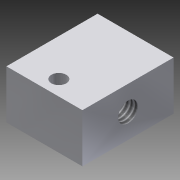
# Autodesk Inventor part: T2.5 belt holder
Saved by Autodesk Inventor 2015 SP1 (Build 190203100, 203)
## iProperties
Created: 2015-04-24
Part Number: T2.5 belt holder
Material: Aluminum 6061
Document SubType Name: Modeling
Designer: ubik
Density: 2.7 g/cm^3
Appearance: Aluminum - Flat
Author: ubik
Autodesk Inventor part; units mm, degrees
ref_plane "YZ Plane" through (0, 0, 0) normal (1, 0, 0) x (0, 1, 0)
ref_plane "XZ Plane" through (0, 0, 0) normal (0, 1, 0) x (-1, 0, 0)
ref_plane "XY Plane" through (0, 0, 0) normal (0, 0, 1) x (1, 0, 0)
sketch "Sketch1" plane through (0, 0, 0) normal (0, 0, 1) x (1, 0, 0)
  line L0 (3.9408, -0.7944) -> (3.5592, -0.7944)
  line L1 (1.4408, -0.7944) -> (1.0592, -0.7944)
  line L2 (-1.0592, -0.7944) -> (-1.4408, -0.7944)
  line L3 (-3.5592, -0.7944) -> (-3.9408, -0.7944)
  line L4 (-6.0592, -0.7944) -> (-6.25, -0.7944)
  line L5 (6.25, -0.7944) -> (6.0592, -0.7944)
  line L6 (6.25, -0.7944) -> (6.25, -8.7944)
  line L7 (6.25, -8.7944) -> (-6.25, -8.7944)
  line L8 (-6.25, -8.7944) -> (-6.25, -0.7944)
  line L9 (-6.25, -0.7944) -> (-6.0592, -0.7944)
  line L10 (-3.9408, -0.7944) -> (-3.5592, -0.7944)
  line L11 (-1.4408, -0.7944) -> (-1.0592, -0.7944)
  line L12 (1.0592, -0.7944) -> (1.4408, -0.7944)
  line L13 (3.5592, -0.7944) -> (3.9408, -0.7944)
  line L14 (6.0592, -0.7944) -> (6.25, -0.7944)
  line L15 (-6.25, -0.7944) -> (6.25, -0.7944)
  point P0 (0, 0)
  dimension "height" = 8
  constraints: 32 end point, 12 horizontal, 7 parallel, 7 perpendicular, 12 other
  measures "height" distance of L6.start L6.end
extrude "Extrusion1" add sketch "Sketch1" against normal blind 15
hole "Hole1" at (-0.125, -8.7944, -2.5) direction (0, 1, 0) diameter 2.459 end through all thread size "M3x0.5" class "6H" standard "ANSI Metric M Profile"
hole "Hole2" at (6.25, -4.7944, -7.5) direction (-1, 0, 0) diameter 3.242 end through all thread size "M4x0.7" class "6H" standard "ANSI Metric M Profile"
equation "\"d12\" = 0.5 * width"
equation "\"d13\" = 0.5 * height"
equation "\"width\" = 15"
body "Solid1"
